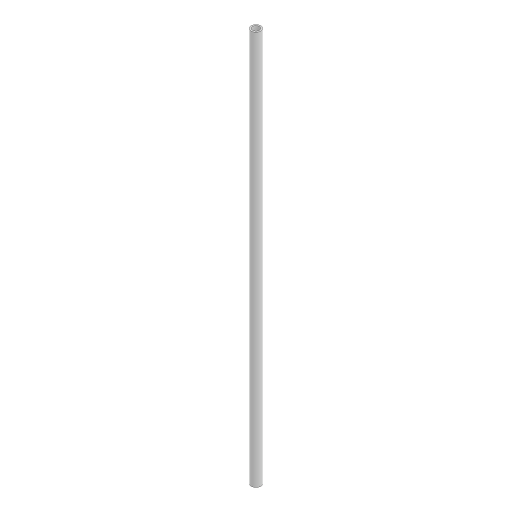
# Autodesk Inventor part: 5P.00.06.01-IB-VTP-Main-Spar
Saved by Autodesk Inventor 2024.3 (Build 283343000, 343)
## iProperties
Created: 2025-01-14
Part Number: 5P.00.06.01-IB-VTP-Main-Spar
Material: Generic
Document SubType Name: Modeling
Designer: inigo
Density: 1 g/cm^3
Appearance: Default
Author: inigo
Autodesk Inventor part; units mm, degrees
ref_plane "YZ Plane" through (0, 0, 0) normal (1, 0, 0) x (0, 1, 0)
ref_plane "XZ Plane" through (0, 0, 0) normal (0, 1, 0) x (-1, 0, 0)
ref_plane "XY Plane" through (0, 0, 0) normal (0, 0, 1) x (1, 0, 0)
sketch "Sketch1" plane through (0, 0, 0) normal (0, 1, 0) x (-1, 0, 0)
  circle A0 centre (0, 0) radius 3.5
  circle A1 centre (0, 0) radius 2.5
  dimension "d0" = 7
  dimension "d3" = 5
  constraints: 2 centre point, 2 coincident
  measures "d0" diameter of A0
  measures "d3" diameter of A1
extrude "Extrusion1" add sketch "Sketch1" along normal blind 285
body "Solid1"
